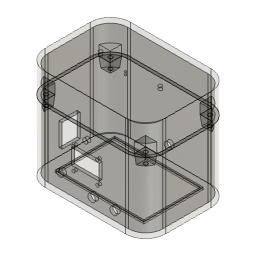
Display_disclosure (Autodesk Fusion 360 design; units mm, degrees)
part number: 2026-03-13-14-21-20-889
Autodesk Fusion 360 part; units mm, degrees
note: some values were not read from the file. Chosen so that the rebuilt part matches the saved one: which bodies a step acts on; which face or edge a step refers to.
sketch "Sketch1" plane through (0, 0, 0) normal (0, 0, 1) x (1, 0, 0)
  line L0 (20, 0) -> (100, 0)
  line L1 (120, 20) -> (120, 65)
  line L2 (100, 85) -> (20, 85)
  line L3 (0, 65) -> (0, 20)
  arc A0 (20, 85) -> (0, 65) centre (20, 65) ccw
  arc A1 (120, 65) -> (100, 85) centre (100, 65) ccw
  arc A2 (100, 0) -> (120, 20) centre (100, 20) ccw
  arc A3 (0, 20) -> (20, 0) centre (20, 20) ccw
  point P0 (120, 0)
  point P1 (0, 85)
  dimension "d1" = 120
  dimension "d2" = 85
  dimension "d3" = 20
  constraint horizontal L0
  constraint vertical L1
  constraint horizontal L2
  constraint vertical L3
  constraint coincident P1 L2
  constraint coincident P1 L3
  constraint tangent L2 A0
  constraint tangent L3 A0
  constraint tangent L1 A1
  constraint tangent L2 A1
  constraint equal A0 A1
  constraint coincident P0 L0
  constraint coincident P0 L1
  constraint tangent L0 A2
  constraint tangent L1 A2
  constraint equal A0 A2
  constraint coincident origin L0
  constraint coincident origin L3
  constraint tangent L0 A3
  constraint tangent L3 A3
  constraint equal A0 A3
  measures "d1" distance of origin P0
  measures "d2" distance of origin P1
  measures "d3" radius of A0
extrude "Extrude1" add sketch "Sketch1" along normal blind 100 makes body 1
shell "Shell1" thickness 3 removed faces 0 bodies 1
sketch "Sketch2" plane through (0, 0, 3) normal (0, 0, 1) x (-1, 0, 0)
  arc A0 (-3, -20) -> (-20, -3) centre (-20, -20) ccw
  line L0 (-20, -3) -> (-100, -3)
  arc A1 (-100, -3) -> (-117, -20) centre (-100, -20) ccw
  line L1 (-117, -20) -> (-117, -65)
  arc A2 (-117, -65) -> (-100, -82) centre (-100, -65) ccw
  line L2 (-100, -82) -> (-20, -82)
  arc A3 (-20, -82) -> (-3, -65) centre (-20, -65) ccw
  line L3 (-3, -65) -> (-3, -20)
  line L4 (-101.8481, -16.4073) -> (-16.8481, -16.4073)
  line L5 (-16.8481, -16.4073) -> (-16.8481, -72.4073)
  line L6 (-16.8481, -72.4073) -> (-101.8481, -72.4073)
  line L7 (-101.8481, -72.4073) -> (-101.8481, -16.4073)
  line L8 (-101.8481, -16.4073) -> (-16.8481, -72.4073) construction
  line L9 (-16.8481, -16.4073) -> (-101.8481, -72.4073) construction
  line L10 (-103.3481, -14.9073) -> (-15.3481, -14.9073)
  line L11 (-15.3481, -14.9073) -> (-15.3481, -73.9073)
  line L12 (-15.3481, -73.9073) -> (-103.3481, -73.9073)
  line L13 (-103.3481, -73.9073) -> (-103.3481, -14.9073)
  point P0 (-59.3481, -44.4073)
  dimension "d7" = 85
  dimension "d8" = 56
  dimension "d9" = -1.5
  constraint horizontal L4
  constraint perpendicular L4 L5
  constraint parallel L4 L6
  constraint parallel L5 L7
  constraint coincident L8 P0
  constraint coincident L9 P0
  measures "d7" distance of L5.end L6.end
  measures "d8" distance of L4.end L5.end
extrude "Extrude2" add sketch "Sketch2" along normal blind 2 contours L10 L11 L12 L13 bodies 1
sketch "Sketch3" plane through (0, 0, 3) normal (0, 0, 1) x (-1, 0, 0)
  arc A0 (-3, -20) -> (-20, -3) centre (-20, -20) ccw
  line L0 (-20, -3) -> (-100, -3)
  arc A1 (-100, -3) -> (-117, -20) centre (-100, -20) ccw
  line L1 (-117, -20) -> (-117, -65)
  arc A2 (-117, -65) -> (-100, -82) centre (-100, -65) ccw
  line L2 (-100, -82) -> (-20, -82)
  arc A3 (-20, -82) -> (-3, -65) centre (-20, -65) ccw
  line L3 (-3, -65) -> (-3, -20)
  line L4 (-103.3481, -73.9073) -> (-103.3481, -14.9073)
  line L5 (-103.3481, -14.9073) -> (-15.3481, -14.9073)
  line L6 (-15.3481, -14.9073) -> (-15.3481, -73.9073)
  line L7 (-15.3481, -73.9073) -> (-103.3481, -73.9073)
  circle A4 centre (-9.1032, -68.8955) radius 3.5
  circle A5 centre (-9.1032, -18.8955) radius 3.5
  circle A6 centre (-9.1032, -68.8955) radius 3.5
  circle A7 centre (-109.1032, -68.8955) radius 3.5
  circle A8 centre (-109.1032, -18.8955) radius 3.5
  circle A9 centre (-109.1032, -18.8955) radius 2
  circle A10 centre (-109.1032, -68.8955) radius 2
  circle A11 centre (-9.1032, -18.8955) radius 2
  circle A12 centre (-9.1032, -68.8955) radius 2
  dimension "d12" = 7
  dimension "d13" = 7
  dimension "d14" = 7
  dimension "d15" = 7
  dimension "d16" = 7
  dimension "d19" = 4
  dimension "d20" = 4
  dimension "d21" = 4
  dimension "d22" = 4
  constraint concentric A8 A9
  constraint concentric A7 A10
  constraint concentric A5 A11
  constraint concentric A4 A12
  measures "d12" diameter of A4
  measures "d13" diameter of A5
  measures "d14" diameter of A6
  measures "d15" diameter of A7
  measures "d16" diameter of A8
  measures "d19" diameter of A9
  measures "d20" diameter of A10
  measures "d21" diameter of A11
  measures "d22" diameter of A12
extrude "Extrude3" add sketch "Sketch3" along normal blind 10 contours A4 A6 | A5 | A7 | A8 | A9 | A10 | A11 | A12 bodies 1
sketch "Sketch4" plane through (0, 0, 3) normal (0, 0, 1) x (-1, 0, 0)
  circle A0 centre (-109.1032, -18.8955) radius 3.5
  circle A1 centre (-109.1032, -68.8955) radius 3.5
  circle A2 centre (-9.1032, -18.8955) radius 3.5
  circle A3 centre (-9.1032, -68.8955) radius 3.5
  arc A4 (-3, -20) -> (-20, -3) centre (-20, -20) ccw
  line L0 (-20, -3) -> (-100, -3)
  arc A5 (-100, -3) -> (-117, -20) centre (-100, -20) ccw
  line L1 (-117, -20) -> (-117, -65)
  arc A6 (-117, -65) -> (-100, -82) centre (-100, -65) ccw
  line L2 (-100, -82) -> (-20, -82)
  arc A7 (-20, -82) -> (-3, -65) centre (-20, -65) ccw
  line L3 (-3, -65) -> (-3, -20)
  line L4 (-103.3481, -73.9073) -> (-103.3481, -14.9073)
  line L5 (-103.3481, -14.9073) -> (-15.3481, -14.9073)
  line L6 (-15.3481, -14.9073) -> (-15.3481, -73.9073)
  line L7 (-15.3481, -73.9073) -> (-103.3481, -73.9073)
extrude "Extrude4" add sketch "Sketch3" along normal blind 70 contours A4 A6 | A5 | A7 | A8 bodies 1
ref_plane "WorkPlane1" through (60, 42.5, 70) normal (0, 0, 1) x (1, 0, 0)
split "Split1" by plane through (60, 42.5, 70) normal (0, 0, 1) bodies 1 makes body 2 at (110.0512, 65.5264, 71) makes body 3 at (73.3333, 28.3333, 100) makes body 4 at (5.6206, 18.547, 71) makes body 5 at (5.8781, 67.536, 71) makes body 6 at (105.6206, 18.547, 71)
delete_body "RemoveBody1" bodies 2
delete_body "RemoveBody2" bodies 5
delete_body "RemoveBody3" bodies 6
delete_body "RemoveBody4" bodies 4
sketch "Sketch5" plane through (0, 0, 100) normal (0, 0, 1) x (-1, 0, 0)
  arc A0 (0, -20) -> (-20, 0) centre (-20, -20) ccw
  line L0 (-20, 0) -> (-100, 0)
  arc A1 (-100, 0) -> (-120, -20) centre (-100, -20) ccw
  line L1 (-120, -20) -> (-120, -65)
  arc A2 (-120, -65) -> (-100, -85) centre (-100, -65) ccw
  line L2 (-100, -85) -> (-20, -85)
  arc A3 (-20, -85) -> (0, -65) centre (-20, -65) ccw
  line L3 (0, -65) -> (0, -20)
sketch "Sketch6" plane through (0, 0, 0) normal (0, -1, 0) x (1, 0, 0)
  line L0 (100, 70) -> (20, 70)
  line L1 (20, 70) -> (20, 0)
  line L2 (20, 0) -> (100, 0)
  line L3 (100, 0) -> (100, 70)
  line L4 (73.75, 32.25) -> (46.25, 32.25)
  line L5 (46.25, 32.25) -> (46.25, 47.75)
  line L6 (46.25, 47.75) -> (73.75, 47.75)
  line L7 (73.75, 47.75) -> (73.75, 32.25)
  line L8 (73.75, 32.25) -> (46.25, 47.75) construction
  line L9 (46.25, 32.25) -> (73.75, 47.75) construction
  line L10 (46.25, 47.75) -> (50.25, 47.75)
  line L11 (73.75, 47.75) -> (69.75, 47.75)
  line L12 (46.25, 32.25) -> (50.25, 32.25)
  line L13 (73.75, 32.25) -> (69.75, 32.25)
  circle A0 centre (34.7701, 19.9292) radius 3.55
  circle A1 centre (66.3615, 14.2033) radius 3.75
  circle A2 centre (88.1009, 13.9302) radius 3.75
  circle A3 centre (48.25, 49.75) radius 1.5
  circle A4 centre (71.75, 49.75) radius 1.5
  circle A5 centre (48.1797, 28.0892) radius 1.5
  circle A6 centre (71.8543, 27.7568) radius 1.5
  point P0 (60, 40)
  dimension "d26" = 27.5
  dimension "d27" = 15.5
  dimension "d28" = 4
  dimension "d30" = 4
  dimension "d32" = 4
  dimension "d34" = 4
  dimension "d40" = 7.1
  dimension "d41" = 7.5
  dimension "d42" = 7.5
  dimension "d43" = 3
  dimension "d44" = 3
  dimension "d45" = 3
  dimension "d46" = 3
  constraint horizontal L4
  constraint perpendicular L4 L5
  constraint parallel L4 L6
  constraint parallel L5 L7
  constraint coincident L8 P0
  constraint coincident L9 P0
  constraint horizontal L10
  constraint horizontal L11
  constraint horizontal L12
  constraint horizontal L13
  measures "d26" distance of L5.end L6.end
  measures "d27" distance of L4.end L5.end
  measures "d28" distance of L5.end L10.end
  measures "d30" distance of L6.end L11.end
  measures "d32" distance of L4.end L12.end
  measures "d34" distance of L4.start L13.end
  measures "d40" diameter of A0
  measures "d41" diameter of A1
  measures "d42" diameter of A2
  measures "d43" diameter of A3
  measures "d44" diameter of A4
  measures "d45" diameter of A5
  measures "d46" diameter of A6
extrude "Extrude5" cut sketch "Sketch6" against normal blind 3 contours L4 L5 L6 L7 L10 L11 L12 L13 | A0 | A1 | A2 | A3 | A4 | A5 | A6 bodies 1
sketch "Sketch7" plane through (0, 0, 100) normal (0, 0, 1) x (-1, 0, 0)
  circle A0 centre (-60.1111, -40.0204) radius 1.05
  circle A1 centre (-30.3411, -45) radius 1.8
  circle A2 centre (-30.3411, -45) radius 1.8
  circle A3 centre (-89.6411, -45) radius 1.8
  dimension "d49" = 2.1
  dimension "d55" = 3.6
  dimension "d56" = 3.6
  dimension "d57" = 3.6
  measures "d49" diameter of A0
  measures "d55" diameter of A1
  measures "d56" diameter of A2
  measures "d57" diameter of A3
extrude "Extrude6" cut sketch "Sketch7" against normal blind 3 bodies 3
sketch "Sketch8" plane through (0, 0, 0) normal (0, -1, 0) x (1, 0, 0)
  circle A0 centre (34.7701, 19.9292) radius 3.55
  circle A1 centre (48.1797, 28.0892) radius 1.5
  circle A2 centre (71.8543, 27.7568) radius 1.5
  circle A3 centre (71.75, 49.75) radius 1.5
  circle A4 centre (88.1009, 13.9302) radius 3.75
  line L0 (46.25, 32.25) -> (46.25, 47.75)
  line L1 (46.25, 47.75) -> (73.75, 47.75)
  line L2 (73.75, 47.75) -> (73.75, 32.25)
  line L3 (73.75, 32.25) -> (46.25, 32.25)
  circle A5 centre (66.3615, 14.2033) radius 3.75
  circle A6 centre (48.25, 49.75) radius 1.5
  line L4 (100, 70) -> (20, 70)
  line L5 (20, 70) -> (20, 0)
  line L6 (20, 0) -> (100, 0)
  line L7 (100, 0) -> (100, 70)
  circle A7 centre (60, 60) radius 2.5
  dimension "d60" = 5
  measures "d60" diameter of A7
extrude "Extrude7" cut sketch "Sketch8" against normal blind 3 contours A7 bodies 1
sketch "Sketch9" plane through (0, 85, 0) normal (0, 1, 0) x (-1, 0, 0)
  line L0 (-20, 70) -> (-100, 70)
  line L1 (-100, 70) -> (-100, 0)
  line L2 (-100, 0) -> (-20, 0)
  line L3 (-20, 0) -> (-20, 70)
  circle A0 centre (-60, 15) radius 3.5
  dimension "d63" = 7
  measures "d63" diameter of A0
extrude "Extrude8" cut sketch "Sketch9" against normal blind 3 contours A0 bodies 1
sketch "Sketch10" plane through (0, 0, 97) normal (0, 0, -1) x (1, 0, 0)
  circle A0 centre (89.6411, -45) radius 1.8
  circle A1 centre (60.1111, -40.0204) radius 1.05
  circle A2 centre (30.3411, -45) radius 1.8
  arc A3 (20, -3) -> (3, -20) centre (20, -20) ccw
  line L0 (3, -20) -> (3, -65)
  arc A4 (3, -65) -> (20, -82) centre (20, -65) ccw
  line L1 (20, -82) -> (100, -82)
  arc A5 (100, -82) -> (117, -65) centre (100, -65) ccw
  line L2 (117, -65) -> (117, -20)
  arc A6 (117, -20) -> (100, -3) centre (100, -20) ccw
  line L3 (100, -3) -> (20, -3)
  circle A7 centre (109, -69) radius 3.5
  circle A8 centre (109, -19) radius 3.5
  circle A9 centre (9, -19) radius 3.5
  circle A10 centre (9, -69) radius 3.5
  circle A11 centre (109, -69) radius 1.95
  circle A12 centre (109, -19) radius 1.95
  circle A13 centre (9, -69) radius 1.95
  circle A14 centre (9, -19) radius 1.95
  dimension "d66" = 7
  dimension "d67" = 7
  dimension "d68" = 7
  dimension "d69" = 7
  dimension "d72" = 3.9
  dimension "d73" = 3.9
  dimension "d74" = 3.9
  dimension "d75" = 3.9
  constraint concentric A7 A11
  constraint concentric A8 A12
  constraint concentric A10 A13
  constraint concentric A9 A14
  measures "d66" diameter of A7
  measures "d67" diameter of A8
  measures "d68" diameter of A9
  measures "d69" diameter of A10
  measures "d72" diameter of A11
  measures "d73" diameter of A12
  measures "d74" diameter of A13
  measures "d75" diameter of A14
extrude "Extrude9" add sketch "Sketch10" along normal blind 5 contours A7 | A8 | A9 | A10 | A11 | A12 | A13 | A14 bodies 3
extrude "Extrude10" add sketch "Sketch10" along normal blind 40 contours A11 | A12 | A13 | A14 bodies 3
sketch "Sketch11" plane through (0, 0, 0) normal (-1, 0, 0) x (0, -1, 0)
  line L0 (-20, 70) -> (-65, 70)
  line L1 (-65, 70) -> (-65, 0)
  line L2 (-65, 0) -> (-20, 0)
  line L3 (-20, 0) -> (-20, 70)
  line L4 (-51.9809, 30.4769) -> (-33.9809, 30.4769)
  line L5 (-33.9809, 30.4769) -> (-33.9809, 7.4769)
  line L6 (-33.9809, 7.4769) -> (-51.9809, 7.4769)
  line L7 (-51.9809, 7.4769) -> (-51.9809, 30.4769)
  dimension "d78" = 18
  constraint horizontal L4
  constraint vertical L5
  constraint horizontal L6
  constraint vertical L7
  measures "d78" distance of L4.start L4.end
extrude "Extrude11" cut sketch "Sketch11" against normal blind 3 contours L4 L5 L6 L7 bodies 1
sketch "Sketch12" plane through (0, 0, 70) normal (0, 0, 1) x (-1, 0, 0)
  line L0 (-3, -20) -> (-3, -65)
  arc A0 (-20, -82) -> (-3, -65) centre (-20, -65) ccw
  line L1 (-20, -82) -> (-100, -82)
  arc A1 (-117, -65) -> (-100, -82) centre (-100, -65) ccw
  line L2 (-117, -65) -> (-117, -20)
  arc A2 (-100, -3) -> (-117, -20) centre (-100, -20) ccw
  line L3 (-100, -3) -> (-20, -3)
  arc A3 (-3, -20) -> (-20, -3) centre (-20, -20) ccw
  line L4 (0, -65) -> (0, -20)
  arc A4 (0, -20) -> (-20, 0) centre (-20, -20) ccw
  line L5 (-20, 0) -> (-100, 0)
  arc A5 (-100, 0) -> (-120, -20) centre (-100, -20) ccw
  line L6 (-120, -20) -> (-120, -65)
  arc A6 (-120, -65) -> (-100, -85) centre (-100, -65) ccw
  line L7 (-100, -85) -> (-20, -85)
  arc A7 (-20, -85) -> (0, -65) centre (-20, -65) ccw
  circle A8 centre (-9.1, -68.9) radius 2
  circle A9 centre (-9.1, -18.9) radius 2
  circle A10 centre (-109.1, -68.9) radius 2
  circle A11 centre (-109.1, -18.9) radius 2
  line L8 (-15, -65) -> (-5, -65)
  line L9 (-5, -65) -> (-5, -75)
  line L10 (-5, -75) -> (-15, -75)
  line L11 (-15, -75) -> (-15, -65)
  line L12 (-15, -15) -> (-5, -15)
  line L13 (-5, -15) -> (-5, -25)
  line L14 (-5, -25) -> (-15, -25)
  line L15 (-15, -25) -> (-15, -15)
  line L16 (-115, -15) -> (-103.781, -15)
  line L17 (-103.781, -15) -> (-103.781, -25)
  line L18 (-103.781, -25) -> (-115, -25)
  line L19 (-115, -25) -> (-115, -15)
  line L20 (-115, -65) -> (-103.781, -65)
  line L21 (-103.781, -65) -> (-103.781, -75.1294)
  line L22 (-103.781, -75.1294) -> (-115, -75.1294)
  line L23 (-115, -75.1294) -> (-115, -65)
  dimension "d83" = 4
  dimension "d84" = 4
  dimension "d85" = 4
  dimension "d86" = 4
  constraint horizontal L8
  constraint vertical L9
  constraint horizontal L10
  constraint vertical L11
  constraint horizontal L12
  constraint vertical L13
  constraint horizontal L14
  constraint vertical L15
  constraint horizontal L16
  constraint vertical L17
  constraint horizontal L18
  constraint vertical L19
  constraint horizontal L20
  constraint vertical L21
  constraint horizontal L22
  constraint vertical L23
  measures "d83" diameter of A8
  measures "d84" diameter of A9
  measures "d85" diameter of A10
  measures "d86" diameter of A11
delete_face "DeleteFace1" 1 faces at (5.8781, 67.536, 47.6667) on bodies 1
delete_face "DeleteFace2" 1 faces at (110.0512, 65.5264, 47.6667) on bodies 1
delete_face "DeleteFace3" 1 faces at (105.6206, 19.244, 25.3333) on bodies 1
delete_face "DeleteFace4" 1 faces at (5.6206, 19.244, 25.3333) on bodies 1
delete_face "DeleteFace5" 2 faces at (10.9403, 18.8058, 80.3333) (9.2375, 18.3949, 57) on bodies 3
delete_face "DeleteFace6" 2 faces at (110.9403, 18.8058, 80.3333) (109.4765, 18.1747, 57) on bodies 3
delete_face "DeleteFace7" 2 faces at (10.3616, 67.6041, 68.6667) (8.7625, 69.6051, 57) on bodies 3
delete_face "DeleteFace8" 2 faces at (110.6639, 67.9832, 80.3333) (109.1446, 70.0169, 57) on bodies 3
delete_face "DeleteFace9" 2 faces at (9.9189, 17.3564, 92) (12.4956, 19.1745, 93.6667) on bodies 3
delete_face "DeleteFace10" 2 faces at (110.1148, 19.3439, 92) (107.8853, 22.3177, 93.6667) on bodies 3
delete_face "DeleteFace11" 2 faces at (107.8852, 68.6561, 92) (107.8853, 72.3177, 93.6667) on bodies 3
delete_face "DeleteFace12" 2 faces at (7.8617, 68.3428, 92) (12.2889, 70.1971, 93.6667) on bodies 3
sketch "Sketch13" plane through (0, 0, 70) normal (0, 0, 1) x (-1, 0, 0)
  line L0 (-3, -20) -> (-3, -65)
  arc A0 (-20, -82) -> (-3, -65) centre (-20, -65) ccw
  line L1 (-20, -82) -> (-100, -82)
  arc A1 (-117, -65) -> (-100, -82) centre (-100, -65) ccw
  line L2 (-117, -65) -> (-117, -20)
  arc A2 (-100, -3) -> (-117, -20) centre (-100, -20) ccw
  line L3 (-100, -3) -> (-20, -3)
  arc A3 (-3, -20) -> (-20, -3) centre (-20, -20) ccw
  line L4 (0, -65) -> (0, -20)
  arc A4 (0, -20) -> (-20, 0) centre (-20, -20) ccw
  line L5 (-20, 0) -> (-100, 0)
  arc A5 (-100, 0) -> (-120, -20) centre (-100, -20) ccw
  line L6 (-120, -20) -> (-120, -65)
  arc A6 (-120, -65) -> (-100, -85) centre (-100, -65) ccw
  line L7 (-100, -85) -> (-20, -85)
  arc A7 (-20, -85) -> (0, -65) centre (-20, -65) ccw
  line L8 (-3.6918, -69.8001) -> (-15, -69.8001)
  line L9 (-15, -69.8001) -> (-15, -81.2481)
  line L10 (-3.7806, -14.9077) -> (-15, -14.9077)
  line L11 (-15, -3.7519) -> (-15, -14.9077)
  line L12 (-104.2301, -81.4653) -> (-104.2301, -70)
  line L13 (-104.2301, -70) -> (-116.2481, -70)
  line L14 (-116.2481, -15) -> (-105, -15)
  line L15 (-105, -15) -> (-105, -3.7519)
  circle A8 centre (-109.3942, -10.7356) radius 2
  circle A9 centre (-109.3942, -74.7356) radius 2
  circle A10 centre (-10.3942, -10.7356) radius 2
  circle A11 centre (-10.3942, -74.7356) radius 2
  dimension "d89" = 4
  dimension "d90" = 4
  dimension "d91" = 4
  dimension "d92" = 4
  constraint coincident A0 L8.start
  constraint horizontal L8
  constraint coincident A0 L9.end
  constraint perpendicular L8 L9
  constraint coincident A3 L10.start
  constraint perpendicular L0 L10
  constraint coincident A3 L11.start
  constraint perpendicular L10 L11
  constraint coincident A1 L12.start
  constraint perpendicular L10 L12
  constraint coincident A1 L13.end
  constraint perpendicular L12 L13
  constraint coincident A2 L14.start
  constraint perpendicular L2 L14
  constraint coincident A2 L15.end
  constraint perpendicular L14 L15
  measures "d89" diameter of A8
  measures "d90" diameter of A9
  measures "d91" diameter of A10
  measures "d92" diameter of A11
extrude "Extrude12" add sketch "Sketch13" against normal blind 10 draft -5 contours A3 L10 L11 | A0 L8 L9 | A2 L14 L15 | A1 L12 L13 | A8 | A9 | A10 | A11 bodies 1
extrude "Extrude13" cut sketch "Sketch13" against normal blind 10 contours A8 | A9 | A10 | A11 bodies 1
sketch "Sketch14" plane through (0, 0, 70) normal (0, 0, -1) x (1, 0, 0)
  line L0 (0, -20) -> (0, -65)
  arc A0 (0, -65) -> (20, -85) centre (20, -65) ccw
  line L1 (20, -85) -> (100, -85)
  arc A1 (100, -85) -> (120, -65) centre (100, -65) ccw
  line L2 (120, -65) -> (120, -20)
  arc A2 (120, -20) -> (100, 0) centre (100, -20) ccw
  line L3 (100, 0) -> (20, 0)
  arc A3 (20, 0) -> (0, -20) centre (20, -20) ccw
  line L4 (3, -65) -> (3, -20)
  arc A4 (20, -3) -> (3, -20) centre (20, -20) ccw
  line L5 (20, -3) -> (100, -3)
  arc A5 (117, -20) -> (100, -3) centre (100, -20) ccw
  line L6 (117, -20) -> (117, -65)
  arc A6 (100, -82) -> (117, -65) centre (100, -65) ccw
  line L7 (100, -82) -> (20, -82)
  arc A7 (3, -65) -> (20, -82) centre (20, -65) ccw
  line L8 (104.0407, -81.5128) -> (104.0407, -70)
  line L9 (104.0407, -70) -> (116.2481, -70)
  line L10 (116.213, -14.8875) -> (105, -14.8875)
  line L11 (105, -14.8875) -> (105, -3.7519)
  line L12 (14.8709, -81.2078) -> (14.8709, -70)
  line L13 (14.8709, -70) -> (3.7519, -70)
  line L14 (3.7519, -15) -> (14.8709, -15)
  line L15 (14.8709, -15) -> (14.8709, -3.7922)
  circle A8 centre (109.3763, -74.7118) radius 1.8
  circle A9 centre (109.3837, -10.7272) radius 1.8
  circle A10 centre (10.3928, -10.7358) radius 1.8
  circle A11 centre (10.3752, -74.7284) radius 1.8
  dimension "d97" = 3.6
  dimension "d98" = 3.6
  dimension "d99" = 3.6
  dimension "d100" = 3.6
  constraint coincident A6 L8.start
  constraint vertical L8
  constraint coincident A6 L9.end
  constraint perpendicular L8 L9
  constraint coincident A5 L10.start
  constraint horizontal L10
  constraint coincident A5 L11.end
  constraint perpendicular L10 L11
  constraint coincident A7 L12.start
  constraint perpendicular L7 L12
  constraint coincident A7 L13.end
  constraint perpendicular L12 L13
  constraint coincident A4 L14.start
  constraint perpendicular L4 L14
  constraint coincident A4 L15.end
  constraint perpendicular L14 L15
  measures "d97" diameter of A8
  measures "d98" diameter of A9
  measures "d99" diameter of A10
  measures "d100" diameter of A11
extrude "Extrude14" add sketch "Sketch14" against normal blind 10 contours A7 L12 L13 | A4 L14 L15 | A6 L8 L9 | A5 L10 L11 | A8 | A9 | A10 | A11 bodies 3
extrude "Extrude15" add sketch "Sketch14" along normal blind 10 contours A8 | A9 | A10 | A11 bodies 3
named bodies: "Body_alarm", "Top_alarm"
